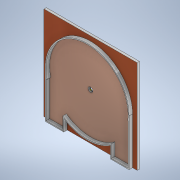
# Autodesk Inventor part: base
Saved by Autodesk Inventor 2021 (Build 250183000, 183)
## iProperties
Created: 2021-07-27
Part Number: base
Material: Aluminum 3004-H32
Document SubType Name: Modeling
Designer: user
Density: 2.71043 g/cm^3
Appearance: Aluminum - Polished
Author: user
Autodesk Inventor part; units mm, degrees
ref_plane "YZ Plane" through (0, 0, 0) normal (1, 0, 0) x (0, 1, 0)
ref_plane "XZ Plane" through (0, 0, 0) normal (0, 1, 0) x (-1, 0, 0)
ref_plane "XY Plane" through (0, 0, 0) normal (0, 0, 1) x (1, 0, 0)
sketch "Sketch1" plane through (0, 0, 0) normal (0, 0, 1) x (1, 0, 0)
  line L0 (10, -10) -> (-10, -10)
  line L1 (-10, -10) -> (-10, 10)
  line L2 (-10, 10) -> (10, 10)
  line L3 (10, 10) -> (10, -10)
  line L4 (10, -10) -> (-10, 10) construction
  line L5 (-10, -10) -> (10, 10) construction
  point P0 (0, 0)
  dimension "d0" = 20
  dimension "d1" = 20
  constraints: 12 end point, 2 midpoint, 2 parallel, 1 horizontal, 1 perpendicular
  measures "d0" distance of L1.end L2.end
  measures "d1" distance of L0.end L1.end
extrude "Extrusion1" add sketch "Sketch1" along normal blind 0.5
sketch "Sketch2" plane through (0, 0, 0.5) normal (0, 0, 1) x (1, 0, 0)
  point P0 (0, 0)
sketch "Sketch3" plane through (0, 0, 0.5) normal (0, 0, 1) x (1, 0, 0)
  line L0 (-10, -10) -> (10, -10) projected
  line L1 (-5, -7.4833) -> (-5, -10)
  line L2 (-5, -10) -> (-9, -10)
  line L3 (-9, -10) -> (-9, 0)
  line L4 (5, 0) -> (9, 0)
  line L5 (9, 0) -> (9, -10)
  line L6 (9, -10) -> (5, -10)
  line L7 (5, -10) -> (5, -7.4833)
  line L8 (-10, 10) -> (-10, -10) projected
  line L9 (10, -10) -> (10, 10) projected
  arc A0 (-5, -7.4833) -> (5, -7.4833) centre (0, 0) ccw
  arc A1 (9, 0) -> (-9, 0) centre (0, 0) ccw
  dimension "d4" = 4
  dimension "d5" = 1
  dimension "d6" = 1
  constraints: 14 end point, 4 point on circle, 3 parallel, 2 centre point, 2 point on line, 1 coincident, 1 horizontal, 1 perpendicular
  measures "d4" distance of L5.end L6.end
  measures "d5" distance between parallel lines of L8 L3
  measures "d6" distance between parallel lines of L9 L5
extrude "Extrusion2" add sketch "Sketch3" along normal blind 0.75 contours L3 A1 L5 L0 L7 A0 L1
sketch "Sketch4" plane through (0, 0, 1.25) normal (0, 0, 1) x (1, 0, 0)
  line L0 (-8.8, -2) -> (-8.5697, -2)
  line L1 (-5.2, -7.0993) -> (-5.2, -9.8)
  line L2 (-5.2, -9.8) -> (-8.8, -9.8)
  line L3 (-8.8, -9.8) -> (-8.8, -2)
  line L4 (-9, 0) -> (-9, -10) projected
  line L5 (-9, -10) -> (-5, -10) projected
  line L6 (-5, -10) -> (-5, -7.4833) projected
  line L7 (8.743, -1) -> (8.8, -1)
  line L8 (8.8, -1) -> (8.8, -9.8)
  line L9 (8.8, -9.8) -> (5.2, -9.8)
  line L10 (5.2, -9.8) -> (5.2, -7.0993)
  line L11 (9, -10) -> (9, 0) projected
  line L12 (5, -10) -> (9, -10) projected
  line L13 (5, -7.4833) -> (5, -10) projected
  arc A0 (-5.2, -7.0993) -> (5.2, -7.0993) centre (0, 0) ccw
  arc A1 (8.743, -1) -> (-8.5697, -2) centre (0, 0) ccw
  dimension "d9" = 0.2
  dimension "d10" = 0.2
  dimension "d11" = 0.2
  dimension "d12" = 0.2
  dimension "d13" = 0.2
  dimension "d14" = 0.2
  constraints: 16 end point, 4 parallel, 4 point on circle, 2 centre point, 2 horizontal, 2 perpendicular, 1 coincident
  measures "d9" distance between parallel lines of L4 L3
  measures "d10" distance between parallel lines of L5 L2
  measures "d11" distance between parallel lines of L6 L1
  measures "d12" distance between parallel lines of L11 L8
  measures "d13" distance between parallel lines of L12 L9
  measures "d14" distance between parallel lines of L13 L10
extrude "Extrusion3" cut sketch "Sketch4" against normal blind 0.75
sketch "Sketch6" plane through (0, 0, 0.5) normal (0, 0, 1) x (1, 0, 0)
  point P0 (0, 0)
sketch "Sketch9" plane through (0, 0, 0.5) normal (0, 0, 1) x (1, 0, 0)
  circle A0 centre (0, 0) radius 0.5
  dimension "d20" = 1
  constraints: 1 centre point, 1 coincident
  measures "d20" diameter of A0
extrude "Extrusion5" cut sketch "Sketch9" against normal blind 0.5
body "Solid1"
